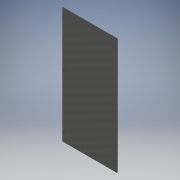
# Autodesk Inventor part: Back PC Cover
Saved by Autodesk Inventor 2019.4 (Build 234330000, 330)
## iProperties
Created: 2020-01-11
Part Number: Back PC Cover
Material: CFRP
Document SubType Name: Modeling
Designer: admin
Density: 1.43 g/cm^3
Appearance: Carbon Fiber
Mass: 530.93 g
Surface Area: 2520.68 cm^2
Volume: 371.28 cm^3
Author: admin
Autodesk Inventor part; units mm, degrees
ref_plane "YZ Plane" through (0, 0, 0) normal (1, 0, 0) x (0, 1, 0)
ref_plane "XZ Plane" through (0, 0, 0) normal (0, 1, 0) x (-1, 0, 0)
ref_plane "XY Plane" through (0, 0, 0) normal (0, 0, 1) x (1, 0, 0)
sketch "Sketch1" plane through (0, 0, 0) normal (0, 0, 1) x (1, 0, 0)
  line L0 (-122, -260) -> (122, -260)
  line L1 (122, -260) -> (122, 260)
  line L2 (122, 260) -> (-122, 260)
  line L3 (-122, 260) -> (-122, -260)
  line L4 (-122, -260) -> (122, 260) construction
  line L5 (122, -260) -> (-122, 260) construction
  point P0 (0, 0)
  dimension "d0" = 244
  dimension "d1" = 520
  constraints: 12 end point, 2 midpoint, 2 parallel, 1 horizontal, 1 perpendicular
  measures "d0" distance of L2.end L1.end
  measures "d1" distance of L1.end L0.end
extrude "Extrusion1" add sketch "Sketch1" along normal blind 3
sketch "Sketch2" plane through (0, 0, 0) normal (0, 0, -1) x (-1, 0, 0)
  circle A0 centre (-110, -219.6952) radius 2.75 projected
  circle A1 centre (-110, 20.3048) radius 2.75 projected
  circle A2 centre (-110, 223.6173) radius 2.75 projected
  circle A3 centre (116, -219.4691) radius 2.75 projected
  circle A4 centre (116, 20.5309) radius 2.75 projected
  circle A5 centre (116, 223.8434) radius 2.75 projected
  point P0 (0, 0)
extrude "Extrusion2" cut sketch "Sketch2" against normal through all
body "Solid1"
